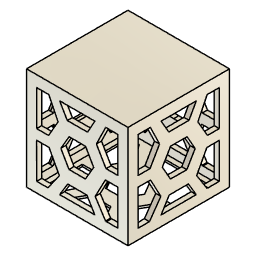
thermal and structural analaysis of cubesat (Autodesk Fusion 360 design; units mm, degrees)
part number: 2025-08-21-17-18-39-864
Autodesk Fusion 360 part; units mm, degrees
sketch "base sketch" plane through (0, 0, 0) normal (0, 0, 1) x (1, 0, 0)
  line L0 (25, -25) -> (-25, -25)
  line L1 (-25, -25) -> (-25, 25)
  line L2 (-25, 25) -> (25, 25)
  line L3 (25, 25) -> (25, -25)
  line L4 (14.1604, 2.5) -> (9.4273, 10.6474)
  line L5 (5.0651, 13.5136) -> (-4.9189, 13.4869)
  line L6 (-9.456, 10.6459) -> (-14.13, 2.5)
  line L7 (-4.6978, -13.5126) -> (4.7384, -13.4873)
  line L8 (8.827, -12.0049) -> (13.8516, -2.5)
  line L9 (8.0828, -0.0479) -> (4.0829, 6.9759)
  line L10 (4.0829, 6.9759) -> (-3.9999, 7.0238)
  line L11 (-3.9999, 7.0238) -> (-8.0828, 0.0479)
  line L12 (-8.0828, 0.0479) -> (-4.0829, -6.9759)
  line L13 (-4.0829, -6.9759) -> (3.9999, -7.0238)
  line L14 (3.9999, -7.0238) -> (8.0828, -0.0479)
  line L15 (-20, 20) -> (-14.435, 20)
  line L16 (-20, 20) -> (-20, 2.5)
  line L17 (-20, -20) -> (-14.435, -20)
  line L18 (-8.691, -20) -> (8.63, -20)
  line L19 (14.404, -20) -> (19.97, -20)
  line L20 (19.97, -20) -> (19.97, -2.5)
  line L21 (19.97, 2.5) -> (19.97, 20)
  line L22 (19.97, 20) -> (14.404, 20)
  line L23 (-8.661, 20) -> (8.66, 20)
  line L24 (8.66, 20) -> (5.0651, 13.5136)
  line L25 (-8.661, 20) -> (-4.9189, 13.4869)
  line L26 (-0.0005, 20) -> (1.3443, 20)
  line L27 (8.63, -20) -> (4.7384, -13.4873)
  line L28 (-8.691, -20) -> (-4.6978, -13.5126)
  line L29 (14, 20) -> (9.4273, 10.6474)
  line L30 (13.9944, 20) -> (16.5751, 20)
  line L31 (19.97, 2.5) -> (14.1604, 2.5)
  line L32 (19.97, -2.5) -> (13.8516, -2.5)
  arc A0 (13.9544, -19.9832) -> (14.404, -20) centre (14.404, -13.9776) ccw
  line L33 (8.827, -12.0049) -> (13.9544, -19.9832)
  line L34 (-14, 20) -> (-9.456, 10.6459)
  line L35 (-14.435, 20) -> (-14, 20)
  line L36 (-20, 2.5) -> (-14.13, 2.5)
  line L37 (-20.03, -20) -> (-20.03, -19.9999)
  line L38 (-20.03, -2.5001) -> (-20.03, -2.5)
  line L39 (-20.03, -20) -> (-20.03, -2.5)
  line L40 (-8.8138, -12.0049) -> (-14.435, -20)
  line L41 (-13.9188, -2.4938) -> (-20.0371, -2.4938)
  line L42 (-13.9188, -2.4938) -> (-8.8138, -12.0049)
  line L43 (-20.03, -2.5) -> (-20, -20)
  line L44 (-20.03, -20) -> (-14.435, -20)
  line L45 (-14.435, -20) -> (-8.8138, -12.0049)
  line L46 (-8.8138, -12.0049) -> (-13.9188, -2.4938)
  line L47 (-20.03, -2.5001) -> (-13.9188, -2.4938)
  line L48 (-13.9188, -2.4938) -> (-8.8138, -12.0049)
  line L49 (-8.8138, -12.0049) -> (-14.435, -20)
  line L50 (-14.435, -20) -> (-20, -20)
  dimension "d1" = 50
  dimension "d2" = 50
  dimension "d9" = 5.565
  dimension "d20" = 17.5
  dimension "d26" = 17.321
  dimension "d28" = 5.566
  dimension "d29" = 17.5
  dimension "d31" = 17.5
  dimension "d32" = 5.566
  dimension "d33" = 17.321
  dimension "d35" = 17.5
  dimension "d36" = 10.7512
  dimension "d37" = 17.5
  constraint horizontal L0
  constraint perpendicular L0 L1
  constraint parallel L0 L2
  constraint parallel L1 L3
  constraint perpendicular L15 L16
  constraint perpendicular L19 L20
  constraint perpendicular L21 L22
  constraint midpoint L23 L26.start
  constraint coincident L23 L26.end
  constraint coincident L22 L30.start
  constraint horizontal L30
  constraint perpendicular L21 L31
  constraint perpendicular L20 L32
  constraint tangent L19 A0
  constraint perpendicular L16 L36
  constraint coincident L38.start L37
  constraint collinear L37 L38
  constraint parallel L17 L44
  constraint perpendicular L39 L50
  measures "d1" distance of L1.end L2.end
  measures "d2" distance of L0.start L2.end
  measures "d9" distance of L15.start L15.end
  measures "d20" distance of L15.start L16.end
  measures "d26" distance of L18.start L18.end
  measures "d28" distance of L19.start L19.end
  measures "d29" distance of L19.end L20.end
  measures "d31" distance of L21.start L21.end
  measures "d32" distance of L21.end L22.end
  measures "d33" distance of L23.start L23.end
  measures "d35" distance of L37.start L38.end
  measures "d36" distance of L8.end L8.start
  measures "d37" distance of L38.end L37.start
extrude "Extrude1" add sketch "base sketch" along normal mid plane 50
sketch "Sketch14" plane through (25, 0, 0) normal (1, 0, 0) x (0, 1, 0)
  line L0 (25, -25) -> (25, 25)
  line L1 (25, 25) -> (-25, 25)
  line L2 (-25, 25) -> (-25, -25)
  line L3 (-25, -25) -> (25, -25)
  line L4 (-8.0828, 0.0479) -> (-4.0829, -6.9759)
  line L5 (8.827, -12.0049) -> (13.8516, -2.5)
  line L6 (-4.6978, -13.5126) -> (4.7384, -13.4873)
  line L7 (19.97, 2.5) -> (19.97, 20)
  line L8 (8.827, -12.0049) -> (13.9544, -19.9832)
  line L9 (8.0828, -0.0479) -> (4.0829, 6.9759)
  line L10 (3.9999, -7.0238) -> (8.0828, -0.0479)
  line L11 (-20, 20) -> (-20, 2.5)
  line L12 (13.9944, 20) -> (16.5751, 20)
  line L13 (-8.661, 20) -> (8.66, 20)
  line L14 (14, 20) -> (9.4273, 10.6474)
  line L15 (-8.691, -20) -> (8.63, -20)
  line L16 (-20, 20) -> (-14.435, 20)
  line L17 (8.63, -20) -> (4.7384, -13.4873)
  line L18 (-9.456, 10.6459) -> (-14.13, 2.5)
  line L19 (14.404, -20) -> (19.97, -20)
  line L20 (-14.435, 20) -> (-14, 20)
  line L21 (-4.0829, -6.9759) -> (3.9999, -7.0238)
  line L22 (14.1604, 2.5) -> (9.4273, 10.6474)
  line L23 (-0.0005, 20) -> (1.3443, 20)
  line L24 (19.97, -20) -> (19.97, -2.5)
  arc A0 (13.9544, -19.9832) -> (14.404, -20) centre (14.404, -13.9776) ccw
  line L25 (8.66, 20) -> (5.0651, 13.5136)
  line L26 (-3.9999, 7.0238) -> (-8.0828, 0.0479)
  line L27 (-13.9188, -2.4938) -> (-8.8138, -12.0049)
  line L28 (19.97, -2.5) -> (13.8516, -2.5)
  line L29 (-20.03, -2.5001) -> (-13.9188, -2.4938)
  line L30 (-20.03, -20) -> (-20.03, -2.5)
  line L31 (19.97, 20) -> (14.404, 20)
  line L32 (4.0829, 6.9759) -> (-3.9999, 7.0238)
  line L33 (-20, 2.5) -> (-14.13, 2.5)
  line L34 (-8.661, 20) -> (-4.9189, 13.4869)
  line L35 (19.97, 2.5) -> (14.1604, 2.5)
  line L36 (-8.8138, -12.0049) -> (-13.9188, -2.4938)
  line L37 (-14, 20) -> (-9.456, 10.6459)
  line L38 (5.0651, 13.5136) -> (-4.9189, 13.4869)
  line L39 (-13.9188, -2.4938) -> (-20.0371, -2.4938)
  line L40 (-8.8138, -12.0049) -> (-14.435, -20)
  line L41 (-20, -20) -> (-14.435, -20)
  line L42 (-20.03, -20) -> (-20.03, -19.9999)
  line L43 (-14.435, -20) -> (-8.8138, -12.0049)
  line L44 (-13.9188, -2.4938) -> (-8.8138, -12.0049)
  line L45 (-20.03, -20) -> (-14.435, -20)
  line L46 (-20.03, -2.5) -> (-20, -20)
  line L47 (-8.8138, -12.0049) -> (-14.435, -20)
  line L48 (-20.03, -2.5001) -> (-20.03, -2.5)
  line L49 (-8.691, -20) -> (-4.6978, -13.5126)
  line L50 (-14.435, -20) -> (-20, -20)
  dimension "d40" = 5.565
  dimension "d41" = 17.5
  dimension "d42" = 17.321
  dimension "d43" = 5.566
  dimension "d44" = 17.5
  dimension "d45" = 17.5
  dimension "d46" = 5.566
  dimension "d47" = 17.321
  dimension "d48" = 17.5
  dimension "d49" = 10.7512
  dimension "d50" = 17.5
  constraint perpendicular L11 L16
  constraint perpendicular L19 L24
  constraint perpendicular L7 L31
  constraint midpoint L23.start L13
  constraint coincident L23.end L13
  constraint coincident L12.start L31
  constraint horizontal L12
  constraint perpendicular L7 L35
  constraint perpendicular L24 L28
  constraint tangent L19 A0
  constraint perpendicular L11 L33
  constraint coincident L29.start L42
  constraint collinear L42 L48
  constraint parallel L41 L45
  constraint perpendicular L30 L50
  measures "d40" distance of L11.start L16.end
  measures "d41" distance of L11.end L11.start
  measures "d42" distance of L15.start L15.end
  measures "d43" distance of L19.start L19.end
  measures "d44" distance of L24.end L19.end
  measures "d45" distance of L7.start L7.end
  measures "d46" distance of L31.end L7.end
  measures "d47" distance of L13.start L13.end
  measures "d48" distance of L30.start L30.end
  measures "d49" distance of L5.start L5.end
  measures "d50" distance of L30.start L30.end
extrude "Extrude2" cut sketch "Sketch14" against normal blind 49 contours L4 L9 L10 L21 L26 L32 | L5 L8 L19 L24 A0 L28 | L6 L15 L17 L49 | L7 L12 L14 L22 L31 L35 | L11 L16 L18 L20 L33 L37 | L13 L23 L25 L34 L38 | L27 L29 L36 L40 L41 L43 L44 L45 L46 L47 L50
sketch "Sketch15" plane through (0, 25, 0) normal (0, 1, 0) x (-1, 0, 0)
  line L0 (25, -25) -> (25, 25)
  line L1 (25, 25) -> (-25, 25)
  line L2 (-25, 25) -> (-25, -25)
  line L3 (-25, -25) -> (25, -25)
  line L4 (-8.0828, 0.0479) -> (-4.0829, -6.9759)
  line L5 (8.827, -12.0049) -> (13.8516, -2.5)
  line L6 (-4.6978, -13.5126) -> (4.7384, -13.4873)
  line L7 (19.97, 2.5) -> (19.97, 20)
  line L8 (8.827, -12.0049) -> (13.9544, -19.9832)
  line L9 (8.0828, -0.0479) -> (4.0829, 6.9759)
  line L10 (3.9999, -7.0238) -> (8.0828, -0.0479)
  line L11 (-20, 20) -> (-20, 2.5)
  line L12 (13.9944, 20) -> (16.5751, 20)
  line L13 (-8.661, 20) -> (8.66, 20)
  line L14 (14, 20) -> (9.4273, 10.6474)
  line L15 (-8.691, -20) -> (8.63, -20)
  line L16 (-20, 20) -> (-14.435, 20)
  line L17 (8.63, -20) -> (4.7384, -13.4873)
  line L18 (-9.456, 10.6459) -> (-14.13, 2.5)
  line L19 (14.404, -20) -> (19.97, -20)
  line L20 (-14.435, 20) -> (-14, 20)
  line L21 (-4.0829, -6.9759) -> (3.9999, -7.0238)
  line L22 (14.1604, 2.5) -> (9.4273, 10.6474)
  line L23 (-0.0005, 20) -> (1.3443, 20)
  line L24 (19.97, -20) -> (19.97, -2.5)
  arc A0 (13.9544, -19.9832) -> (14.404, -20) centre (14.404, -13.9776) ccw
  line L25 (8.66, 20) -> (5.0651, 13.5136)
  line L26 (-3.9999, 7.0238) -> (-8.0828, 0.0479)
  line L27 (-13.9188, -2.4938) -> (-8.8138, -12.0049)
  line L28 (19.97, -2.5) -> (13.8516, -2.5)
  line L29 (-20.03, -2.5001) -> (-13.9188, -2.4938)
  line L30 (-20.03, -20) -> (-20.03, -2.5)
  line L31 (19.97, 20) -> (14.404, 20)
  line L32 (4.0829, 6.9759) -> (-3.9999, 7.0238)
  line L33 (-20, 2.5) -> (-14.13, 2.5)
  line L34 (-8.661, 20) -> (-4.9189, 13.4869)
  line L35 (19.97, 2.5) -> (14.1604, 2.5)
  line L36 (-8.8138, -12.0049) -> (-13.9188, -2.4938)
  line L37 (-14, 20) -> (-9.456, 10.6459)
  line L38 (5.0651, 13.5136) -> (-4.9189, 13.4869)
  line L39 (-13.9188, -2.4938) -> (-20.0371, -2.4938)
  line L40 (-8.8138, -12.0049) -> (-14.435, -20)
  line L41 (-20, -20) -> (-14.435, -20)
  line L42 (-20.03, -20) -> (-20.03, -19.9999)
  line L43 (-14.435, -20) -> (-8.8138, -12.0049)
  line L44 (-13.9188, -2.4938) -> (-8.8138, -12.0049)
  line L45 (-20.03, -20) -> (-14.435, -20)
  line L46 (-20.03, -2.5) -> (-20, -20)
  line L47 (-8.8138, -12.0049) -> (-14.435, -20)
  line L48 (-20.03, -2.5001) -> (-20.03, -2.5)
  line L49 (-8.691, -20) -> (-4.6978, -13.5126)
  line L50 (-14.435, -20) -> (-20, -20)
  dimension "d53" = 5.565
  dimension "d54" = 17.5
  dimension "d55" = 17.321
  dimension "d56" = 5.566
  dimension "d57" = 17.5
  dimension "d58" = 17.5
  dimension "d59" = 5.566
  dimension "d60" = 17.321
  dimension "d61" = 17.5
  dimension "d62" = 10.7512
  dimension "d63" = 17.5
  constraint perpendicular L11 L16
  constraint perpendicular L19 L24
  constraint perpendicular L7 L31
  constraint midpoint L23.start L13
  constraint coincident L23.end L13
  constraint coincident L12.start L31
  constraint horizontal L12
  constraint perpendicular L7 L35
  constraint perpendicular L24 L28
  constraint tangent L19 A0
  constraint perpendicular L11 L33
  constraint coincident L29.start L42
  constraint collinear L42 L48
  constraint parallel L41 L45
  constraint perpendicular L30 L50
  measures "d53" distance of L11.start L16.end
  measures "d54" distance of L11.end L11.start
  measures "d55" distance of L15.start L15.end
  measures "d56" distance of L19.start L19.end
  measures "d57" distance of L24.end L19.end
  measures "d58" distance of L7.start L7.end
  measures "d59" distance of L31.end L7.end
  measures "d60" distance of L13.start L13.end
  measures "d61" distance of L30.start L30.end
  measures "d62" distance of L5.start L5.end
  measures "d63" distance of L30.start L30.end
extrude "Extrude3" cut sketch "Sketch15" against normal blind 25 contours L4 L9 L10 L21 L26 L32 | L5 L8 L19 L24 A0 L28 | L6 L15 L17 L49 | L7 L12 L14 L22 L31 L35 | L11 L16 L18 L20 L33 L37 | L13 L23 L25 L34 L38 | L27 L29 L36 L40 L41 L43 L44 L45 L46 L47 L50
sketch "Sketch16" plane through (0, -25, 0) normal (0, -1, 0) x (1, 0, 0)
  line L0 (25, -25) -> (25, 25)
  line L1 (25, 25) -> (-25, 25)
  line L2 (-25, 25) -> (-25, -25)
  line L3 (-25, -25) -> (25, -25)
  line L4 (-8.0828, 0.0479) -> (-4.0829, -6.9759)
  line L5 (8.827, -12.0049) -> (13.8516, -2.5)
  line L6 (-4.6978, -13.5126) -> (4.7384, -13.4873)
  line L7 (19.97, 2.5) -> (19.97, 20)
  line L8 (8.827, -12.0049) -> (13.9544, -19.9832)
  line L9 (8.0828, -0.0479) -> (4.0829, 6.9759)
  line L10 (3.9999, -7.0238) -> (8.0828, -0.0479)
  line L11 (-20, 20) -> (-20, 2.5)
  line L12 (13.9944, 20) -> (16.5751, 20)
  line L13 (-8.661, 20) -> (8.66, 20)
  line L14 (14, 20) -> (9.4273, 10.6474)
  line L15 (-8.691, -20) -> (8.63, -20)
  line L16 (-20, 20) -> (-14.435, 20)
  line L17 (8.63, -20) -> (4.7384, -13.4873)
  line L18 (-9.456, 10.6459) -> (-14.13, 2.5)
  line L19 (14.404, -20) -> (19.97, -20)
  line L20 (-14.435, 20) -> (-14, 20)
  line L21 (-4.0829, -6.9759) -> (3.9999, -7.0238)
  line L22 (14.1604, 2.5) -> (9.4273, 10.6474)
  line L23 (-0.0005, 20) -> (1.3443, 20)
  line L24 (19.97, -20) -> (19.97, -2.5)
  arc A0 (13.9544, -19.9832) -> (14.404, -20) centre (14.404, -13.9776) ccw
  line L25 (8.66, 20) -> (5.0651, 13.5136)
  line L26 (-3.9999, 7.0238) -> (-8.0828, 0.0479)
  line L27 (-13.9188, -2.4938) -> (-8.8138, -12.0049)
  line L28 (19.97, -2.5) -> (13.8516, -2.5)
  line L29 (-20.03, -2.5001) -> (-13.9188, -2.4938)
  line L30 (-20.03, -20) -> (-20.03, -2.5)
  line L31 (19.97, 20) -> (14.404, 20)
  line L32 (4.0829, 6.9759) -> (-3.9999, 7.0238)
  line L33 (-20, 2.5) -> (-14.13, 2.5)
  line L34 (-8.661, 20) -> (-4.9189, 13.4869)
  line L35 (19.97, 2.5) -> (14.1604, 2.5)
  line L36 (-8.8138, -12.0049) -> (-13.9188, -2.4938)
  line L37 (-14, 20) -> (-9.456, 10.6459)
  line L38 (5.0651, 13.5136) -> (-4.9189, 13.4869)
  line L39 (-13.9188, -2.4938) -> (-20.0371, -2.4938)
  line L40 (-8.8138, -12.0049) -> (-14.435, -20)
  line L41 (-20, -20) -> (-14.435, -20)
  line L42 (-20.03, -20) -> (-20.03, -19.9999)
  line L43 (-14.435, -20) -> (-8.8138, -12.0049)
  line L44 (-13.9188, -2.4938) -> (-8.8138, -12.0049)
  line L45 (-20.03, -20) -> (-14.435, -20)
  line L46 (-20.03, -2.5) -> (-20, -20)
  line L47 (-8.8138, -12.0049) -> (-14.435, -20)
  line L48 (-20.03, -2.5001) -> (-20.03, -2.5)
  line L49 (-8.691, -20) -> (-4.6978, -13.5126)
  line L50 (-14.435, -20) -> (-20, -20)
  dimension "d66" = 5.565
  dimension "d67" = 17.5
  dimension "d68" = 17.321
  dimension "d69" = 5.566
  dimension "d70" = 17.5
  dimension "d71" = 17.5
  dimension "d72" = 5.566
  dimension "d73" = 17.321
  dimension "d74" = 17.5
  dimension "d75" = 10.7512
  dimension "d76" = 17.5
  constraint perpendicular L11 L16
  constraint perpendicular L19 L24
  constraint perpendicular L7 L31
  constraint midpoint L23.start L13
  constraint coincident L23.end L13
  constraint coincident L12.start L31
  constraint horizontal L12
  constraint perpendicular L7 L35
  constraint perpendicular L24 L28
  constraint tangent L19 A0
  constraint perpendicular L11 L33
  constraint coincident L29.start L42
  constraint collinear L42 L48
  constraint parallel L41 L45
  constraint perpendicular L30 L50
  measures "d66" distance of L11.start L16.end
  measures "d67" distance of L11.end L11.start
  measures "d68" distance of L15.start L15.end
  measures "d69" distance of L19.start L19.end
  measures "d70" distance of L24.end L19.end
  measures "d71" distance of L7.start L7.end
  measures "d72" distance of L31.end L7.end
  measures "d73" distance of L13.start L13.end
  measures "d74" distance of L30.start L30.end
  measures "d75" distance of L5.start L5.end
  measures "d76" distance of L30.start L30.end
extrude "Extrude4" cut sketch "Sketch16" against normal blind 50 contours L4 L9 L10 L21 L26 L32 | L5 L8 L19 L24 A0 L28 | L6 L15 L17 L49 | L7 L12 L14 L22 L31 L35 | L11 L16 L18 L20 L33 L37 | L13 L23 L25 L34 L38 | L27 L29 L36 L40 L41 L43 L44 L45 L46 L47 L50
sketch "Sketch17" plane through (-25, 0, 0) normal (-1, 0, 0) x (0, -1, 0)
  line L0 (25, -25) -> (25, 25)
  line L1 (25, 25) -> (-25, 25)
  line L2 (-25, 25) -> (-25, -25)
  line L3 (-25, -25) -> (25, -25)
  line L4 (-8.0828, 0.0479) -> (-4.0829, -6.9759)
  line L5 (8.827, -12.0049) -> (13.8516, -2.5)
  line L6 (-4.6978, -13.5126) -> (4.7384, -13.4873)
  line L7 (19.97, 2.5) -> (19.97, 20)
  line L8 (8.827, -12.0049) -> (13.9544, -19.9832)
  line L9 (8.0828, -0.0479) -> (4.0829, 6.9759)
  line L10 (3.9999, -7.0238) -> (8.0828, -0.0479)
  line L11 (-20, 20) -> (-20, 2.5)
  line L12 (13.9944, 20) -> (16.5751, 20)
  line L13 (-8.661, 20) -> (8.66, 20)
  line L14 (14, 20) -> (9.4273, 10.6474)
  line L15 (-8.691, -20) -> (8.63, -20)
  line L16 (-20, 20) -> (-14.435, 20)
  line L17 (8.63, -20) -> (4.7384, -13.4873)
  line L18 (-9.456, 10.6459) -> (-14.13, 2.5)
  line L19 (14.404, -20) -> (19.97, -20)
  line L20 (-14.435, 20) -> (-14, 20)
  line L21 (-4.0829, -6.9759) -> (3.9999, -7.0238)
  line L22 (14.1604, 2.5) -> (9.4273, 10.6474)
  line L23 (-0.0005, 20) -> (1.3443, 20)
  line L24 (19.97, -20) -> (19.97, -2.5)
  arc A0 (13.9544, -19.9832) -> (14.404, -20) centre (14.404, -13.9776) ccw
  line L25 (8.66, 20) -> (5.0651, 13.5136)
  line L26 (-3.9999, 7.0238) -> (-8.0828, 0.0479)
  line L27 (-13.9188, -2.4938) -> (-8.8138, -12.0049)
  line L28 (19.97, -2.5) -> (13.8516, -2.5)
  line L29 (-20.03, -2.5001) -> (-13.9188, -2.4938)
  line L30 (-20.03, -20) -> (-20.03, -2.5)
  line L31 (19.97, 20) -> (14.404, 20)
  line L32 (4.0829, 6.9759) -> (-3.9999, 7.0238)
  line L33 (-20, 2.5) -> (-14.13, 2.5)
  line L34 (-8.661, 20) -> (-4.9189, 13.4869)
  line L35 (19.97, 2.5) -> (14.1604, 2.5)
  line L36 (-8.8138, -12.0049) -> (-13.9188, -2.4938)
  line L37 (-14, 20) -> (-9.456, 10.6459)
  line L38 (5.0651, 13.5136) -> (-4.9189, 13.4869)
  line L39 (-13.9188, -2.4938) -> (-20.0371, -2.4938)
  line L40 (-8.8138, -12.0049) -> (-14.435, -20)
  line L41 (-20, -20) -> (-14.435, -20)
  line L42 (-20.03, -20) -> (-20.03, -19.9999)
  line L43 (-14.435, -20) -> (-8.8138, -12.0049)
  line L44 (-13.9188, -2.4938) -> (-8.8138, -12.0049)
  line L45 (-20.03, -20) -> (-14.435, -20)
  line L46 (-20.03, -2.5) -> (-20, -20)
  line L47 (-8.8138, -12.0049) -> (-14.435, -20)
  line L48 (-20.03, -2.5001) -> (-20.03, -2.5)
  line L49 (-8.691, -20) -> (-4.6978, -13.5126)
  line L50 (-14.435, -20) -> (-20, -20)
  dimension "d79" = 5.565
  dimension "d80" = 17.5
  dimension "d81" = 17.321
  dimension "d82" = 5.566
  dimension "d83" = 17.5
  dimension "d84" = 17.5
  dimension "d85" = 5.566
  dimension "d86" = 17.321
  dimension "d87" = 17.5
  dimension "d88" = 10.7512
  dimension "d89" = 17.5
  constraint perpendicular L11 L16
  constraint perpendicular L19 L24
  constraint perpendicular L7 L31
  constraint midpoint L23.start L13
  constraint coincident L23.end L13
  constraint coincident L12.start L31
  constraint horizontal L12
  constraint perpendicular L7 L35
  constraint perpendicular L24 L28
  constraint tangent L19 A0
  constraint perpendicular L11 L33
  constraint coincident L29.start L42
  constraint collinear L42 L48
  constraint parallel L41 L45
  constraint perpendicular L30 L50
  measures "d79" distance of L11.start L16.end
  measures "d80" distance of L11.end L11.start
  measures "d81" distance of L15.start L15.end
  measures "d82" distance of L19.start L19.end
  measures "d83" distance of L24.end L19.end
  measures "d84" distance of L7.start L7.end
  measures "d85" distance of L31.end L7.end
  measures "d86" distance of L13.start L13.end
  measures "d87" distance of L30.start L30.end
  measures "d88" distance of L5.start L5.end
  measures "d89" distance of L30.start L30.end
extrude "Extrude5" cut sketch "Sketch17" against normal blind 1 contours L4 L9 L10 L21 L26 L32 | L5 L8 L19 L24 A0 L28 | L6 L15 L17 L49 | L7 L12 L14 L22 L31 L35 | L11 L16 L18 L20 L33 L37 | L13 L23 L25 L34 L38 | L27 L29 L36 L40 L41 L43 L44 L45 L46 L47 L50
sketch "Sketch18" plane through (0, 0, 25) normal (0, 0, 1) x (-1, 0, 0)
  line L0 (-13.9544, 19.9832) -> (-8.827, 12.0049)
  line L1 (-8.827, 12.0049) -> (-13.8516, 2.5)
  line L2 (-13.8516, 2.5) -> (-19.97, 2.5)
  line L3 (-19.97, 2.5) -> (-19.97, 20)
  line L4 (-19.97, 20) -> (-14.404, 20)
  arc A0 (-13.9544, 19.9832) -> (-14.404, 20) centre (-14.404, 13.9776) ccw
  line L5 (-8.0828, 0.0479) -> (-3.9999, 7.0238)
  line L6 (-3.9999, 7.0238) -> (4.0829, 6.9759)
  line L7 (4.0829, 6.9759) -> (8.0828, -0.0479)
  line L8 (8.0828, -0.0479) -> (3.9999, -7.0238)
  line L9 (3.9999, -7.0238) -> (-4.0829, -6.9759)
  line L10 (-4.0829, -6.9759) -> (-8.0828, 0.0479)
  line L11 (8.8138, 12.0049) -> (14.435, 20)
  line L12 (14.435, 20) -> (20.03, 20)
  line L13 (20.03, 20) -> (20.03, 2.5001)
  line L14 (20.03, 2.5001) -> (13.9188, 2.4938)
  line L15 (13.9188, 2.4938) -> (8.8138, 12.0049)
  line L16 (-4.7384, 13.4873) -> (-8.63, 20)
  line L17 (-8.63, 20) -> (8.691, 20)
  line L18 (8.691, 20) -> (4.6978, 13.5126)
  line L19 (4.6978, 13.5126) -> (-4.7384, 13.4873)
  line L20 (20, -2.5) -> (20, -20)
  line L21 (20, -20) -> (14.435, -20)
  line L22 (14.435, -20) -> (14, -20)
  line L23 (14, -20) -> (9.456, -10.6459)
  line L24 (9.456, -10.6459) -> (14.13, -2.5)
  line L25 (14.13, -2.5) -> (20, -2.5)
  line L26 (4.9189, -13.4869) -> (8.661, -20)
  line L27 (8.661, -20) -> (-8.66, -20)
  line L28 (-8.66, -20) -> (-5.0651, -13.5136)
  line L29 (-5.0651, -13.5136) -> (4.9189, -13.4869)
  line L30 (-14, -20) -> (-19.97, -20)
  line L31 (-19.97, -20) -> (-19.97, -2.5)
  line L32 (-19.97, -2.5) -> (-14.1604, -2.5)
  line L33 (-14.1604, -2.5) -> (-9.4273, -10.6474)
  line L34 (-9.4273, -10.6474) -> (-14, -20)
  line L35 (-25, -25) -> (25, -25)
  line L36 (25, -25) -> (25, 25)
  line L37 (25, 25) -> (-25, 25)
  line L38 (-25, 25) -> (-25, -25)
  line L39 (-25, 25) -> (25, 25)
  line L40 (25, 25) -> (25, -25)
  line L41 (25, -25) -> (-25, -25)
  line L42 (-25, -25) -> (-25, 25)
  line L43 (-25, 25) -> (25, -25) construction
  line L44 (25, 25) -> (-25, -25) construction
  constraint horizontal L39
  constraint perpendicular L39 L40
  constraint parallel L39 L41
  constraint parallel L40 L42
  constraint coincident L43 origin
  constraint coincident L44 origin
  constraint coincident L37.end L38.start
extrude "Extrude6" add sketch "Sketch18" along normal blind 0.5 contours L0 L1 L2 L3 L4 A0 | L5 L6 L7 L8 L9 L10 | L11 L12 L13 L14 L15 | L16 L17 L18 L19 | L20 L21 L22 L23 L24 L25 | L26 L27 L28 L29 | L30 L31 L32 L33 L34 | L35 L36 L37 L38 L39 L40 L41 L42
sketch "Sketch19" plane through (25, 0, 0) normal (1, 0, 0) x (0, 1, 0)
sketch "Sketch20" plane through (0, 0, -25) normal (0, 0, -1) x (1, 0, 0)
  line L0 (8.827, 12.0049) -> (13.9544, 19.9832)
  arc A0 (14.404, 20) -> (13.9544, 19.9832) centre (14.404, 13.9776) ccw
  line L1 (14.404, 20) -> (19.97, 20)
  line L2 (19.97, 20) -> (19.97, 2.5)
  line L3 (19.97, 2.5) -> (13.8516, 2.5)
  line L4 (13.8516, 2.5) -> (8.827, 12.0049)
  line L5 (3.9999, 7.0238) -> (8.0828, 0.0479)
  line L6 (8.0828, 0.0479) -> (4.0829, -6.9759)
  line L7 (4.0829, -6.9759) -> (-3.9999, -7.0238)
  line L8 (-3.9999, -7.0238) -> (-8.0828, -0.0479)
  line L9 (-8.0828, -0.0479) -> (-4.0829, 6.9759)
  line L10 (-4.0829, 6.9759) -> (3.9999, 7.0238)
  line L11 (-14.435, 20) -> (-8.8138, 12.0049)
  line L12 (-8.8138, 12.0049) -> (-13.9188, 2.4938)
  line L13 (-13.9188, 2.4938) -> (-20.03, 2.5001)
  line L14 (-20.03, 2.5001) -> (-20.03, 20)
  line L15 (-20.03, 20) -> (-14.435, 20)
  line L16 (8.63, 20) -> (4.7384, 13.4873)
  line L17 (4.7384, 13.4873) -> (-4.6978, 13.5126)
  line L18 (-4.6978, 13.5126) -> (-8.691, 20)
  line L19 (-8.691, 20) -> (8.63, 20)
  line L20 (-20, -20) -> (-20, -2.5)
  line L21 (-20, -2.5) -> (-14.13, -2.5)
  line L22 (-14.13, -2.5) -> (-9.456, -10.6459)
  line L23 (-9.456, -10.6459) -> (-14, -20)
  line L24 (-14, -20) -> (-14.435, -20)
  line L25 (-14.435, -20) -> (-20, -20)
  line L26 (-8.661, -20) -> (-4.9189, -13.4869)
  line L27 (-4.9189, -13.4869) -> (5.0651, -13.5136)
  line L28 (5.0651, -13.5136) -> (8.66, -20)
  line L29 (8.66, -20) -> (-8.661, -20)
  line L30 (19.97, -20) -> (14, -20)
  line L31 (14, -20) -> (9.4273, -10.6474)
  line L32 (9.4273, -10.6474) -> (14.1604, -2.5)
  line L33 (14.1604, -2.5) -> (19.97, -2.5)
  line L34 (19.97, -2.5) -> (19.97, -20)
  line L35 (-25, -25) -> (25, -25)
  line L36 (25, -25) -> (25, 25)
  line L37 (25, 25) -> (-25, 25)
  line L38 (-25, 25) -> (-25, -25)
  line L39 (22.5, 22.5) -> (-22.5, 22.5)
  line L40 (-22.5, 22.5) -> (-22.5, -22.5)
  line L41 (-22.5, -22.5) -> (22.5, -22.5)
  line L42 (22.5, -22.5) -> (22.5, 22.5)
  line L43 (22.5, 22.5) -> (-22.5, -22.5) construction
  line L44 (-22.5, 22.5) -> (22.5, -22.5) construction
  dimension "d94" = 45
  dimension "d95" = 45
  constraint horizontal L39
  constraint perpendicular L39 L40
  constraint parallel L39 L41
  constraint parallel L40 L42
  constraint coincident L43 origin
  constraint coincident L44 origin
  measures "d94" distance of L40.end L41.end
  measures "d95" distance of L39.end L40.end
ref_plane "WorkPlane1" through (0, 0, -24) normal (0, 0, -1) x (1, 0, 0)
extrude "Extrude7" cut sketch "Sketch20" against normal blind 48 contours L39 L40 L41 L42
sketch "Sketch21" plane through (25, 0, 0) normal (1, 0, 0) x (0, 1, 0)
sketch "Sketch22" plane through (0, 0, -25) normal (0, 0, -1) x (1, 0, 0)
  line L0 (-22.5, 22.5) -> (22.5, 22.5)
  line L1 (22.5, 22.5) -> (22.5, -22.5)
  line L2 (22.5, -22.5) -> (-22.5, -22.5)
  line L3 (-22.5, -22.5) -> (-22.5, 22.5)
  line L4 (-25, -25) -> (25, -25)
  line L5 (25, -25) -> (25, 25)
  line L6 (25, 25) -> (-25, 25)
  line L7 (-25, 25) -> (-25, -25)
  line L8 (25, -25) -> (-25, -25)
  line L9 (-25, -25) -> (-25, 25)
  line L10 (-25, 25) -> (25, 25)
  line L11 (25, 25) -> (25, -25)
  line L12 (25, -25) -> (-25, 25) construction
  line L13 (-25, -25) -> (25, 25) construction
  constraint horizontal L8
  constraint perpendicular L8 L9
  constraint parallel L8 L10
  constraint parallel L9 L11
  constraint coincident L12 origin
  constraint coincident L13 origin
  constraint coincident L4.end L5.start
sketch "Sketch23" plane through (0, 0, -25) normal (0, 0, -1) x (1, 0, 0)
sketch "Sketch24" plane through (0, 0, 0) normal (0, 0, 1) x (1, 0, 0)
  line L0 (-25, -25) -> (25, -25)
  line L1 (25, -25) -> (25, 25)
  line L2 (25, 25) -> (-25, 25)
  line L3 (-25, 25) -> (-25, -25)
  line L4 (-25, -25) -> (25, 25) construction
  line L5 (25, -25) -> (-25, 25) construction
  line L6 (19.97, -2.5) -> (13.8516, -2.5)
  line L7 (-13.9188, -2.4938) -> (-8.8138, -12.0049)
  line L8 (-20.03, -20) -> (-20.03, -19.9999)
  line L9 (-13.9188, -2.4938) -> (-20.0371, -2.4938)
  line L10 (-0.0005, 20) -> (1.3443, 20)
  line L11 (-20, -20) -> (-14.435, -20)
  line L12 (-8.8138, -12.0049) -> (-14.435, -20)
  arc A0 (13.9544, -19.9832) -> (14.404, -20) centre (14.404, -13.9776) ccw
  line L13 (8.63, -20) -> (4.7384, -13.4873)
  line L14 (-3.9999, 7.0238) -> (-8.0828, 0.0479)
  line L15 (19.97, -20) -> (19.97, -2.5)
  line L16 (14, 20) -> (9.4273, 10.6474)
  line L17 (-8.691, -20) -> (-4.6978, -13.5126)
  line L18 (14.1604, 2.5) -> (9.4273, 10.6474)
  line L19 (-8.661, 20) -> (-4.9189, 13.4869)
  line L20 (-9.456, 10.6459) -> (-14.13, 2.5)
  line L21 (-20, 20) -> (-20, 2.5)
  line L22 (-14.435, 20) -> (-14, 20)
  line L23 (8.66, 20) -> (5.0651, 13.5136)
  line L24 (-20.03, -2.5001) -> (-13.9188, -2.4938)
  line L25 (-8.8138, -12.0049) -> (-14.435, -20)
  line L26 (-14.435, -20) -> (-8.8138, -12.0049)
  line L27 (8.827, -12.0049) -> (13.9544, -19.9832)
  line L28 (-8.661, 20) -> (8.66, 20)
  line L29 (-14.435, -20) -> (-20, -20)
  line L30 (8.827, -12.0049) -> (13.8516, -2.5)
  line L31 (4.0829, 6.9759) -> (-3.9999, 7.0238)
  line L32 (13.9944, 20) -> (16.5751, 20)
  line L33 (14.404, -20) -> (19.97, -20)
  line L34 (19.97, 2.5) -> (19.97, 20)
  line L35 (5.0651, 13.5136) -> (-4.9189, 13.4869)
  line L36 (8.0828, -0.0479) -> (4.0829, 6.9759)
  line L37 (-8.0828, 0.0479) -> (-4.0829, -6.9759)
  line L38 (-4.0829, -6.9759) -> (3.9999, -7.0238)
  line L39 (-4.6978, -13.5126) -> (4.7384, -13.4873)
  line L40 (-8.691, -20) -> (8.63, -20)
  line L41 (3.9999, -7.0238) -> (8.0828, -0.0479)
  line L42 (-20, 20) -> (-14.435, 20)
  line L43 (-13.9188, -2.4938) -> (-8.8138, -12.0049)
  line L44 (-20, 2.5) -> (-14.13, 2.5)
  line L45 (-20.03, -20) -> (-20.03, -2.5)
  line L46 (-14, 20) -> (-9.456, 10.6459)
  line L47 (-20.03, -2.5001) -> (-20.03, -2.5)
  line L48 (-20.03, -20) -> (-14.435, -20)
  line L49 (19.97, 2.5) -> (14.1604, 2.5)
  line L50 (-20.03, -2.5) -> (-20, -20)
  line L51 (19.97, 20) -> (14.404, 20)
  line L52 (-8.8138, -12.0049) -> (-13.9188, -2.4938)
  dimension "d99" = 5.565
  dimension "d100" = 17.5
  dimension "d101" = 17.321
  dimension "d102" = 5.566
  dimension "d103" = 17.5
  dimension "d104" = 17.5
  dimension "d105" = 5.566
  dimension "d106" = 17.321
  dimension "d107" = 17.5
  dimension "d108" = 10.7512
  dimension "d109" = 17.5
  constraint horizontal L0
  constraint perpendicular L0 L1
  constraint parallel L0 L2
  constraint parallel L1 L3
  constraint coincident L4 origin
  constraint coincident L5 origin
  constraint perpendicular L21 L42
  constraint perpendicular L15 L33
  constraint perpendicular L34 L51
  constraint midpoint L10.start L28
  constraint coincident L10.end L28
  constraint coincident L32.start L51
  constraint horizontal L32
  constraint perpendicular L34 L49
  constraint perpendicular L6 L15
  constraint tangent A0 L33
  constraint perpendicular L21 L44
  constraint coincident L24.start L8
  constraint collinear L8 L47
  constraint parallel L11 L48
  constraint perpendicular L29 L45
  measures "d99" distance of L21.start L22.start
  measures "d100" distance of L21.end L21.start
  measures "d101" distance of L17.start L13.start
  measures "d102" distance of L15.start A0.end
  measures "d103" distance of L15.start L6.start
  measures "d104" distance of L34.end L34.start
  measures "d105" distance of L51.end L34.end
  measures "d106" distance of L19.start L23.start
  measures "d107" distance of L45.end L8.start
  measures "d108" distance of L27.start L6.end
  measures "d109" distance of L8.start L45.end
sketch "Sketch25" plane through (0, 0, 0) normal (0, 0, 1) x (1, 0, 0)
  line L0 (-25, -25) -> (25, -25)
  line L1 (25, -25) -> (25, 25)
  line L2 (25, 25) -> (-25, 25)
  line L3 (-25, 25) -> (-25, -25)
  line L4 (-25, -25) -> (25, 25) construction
  line L5 (25, -25) -> (-25, 25) construction
  constraint horizontal L0
  constraint perpendicular L0 L1
  constraint parallel L0 L2
  constraint parallel L1 L3
  constraint coincident L4 origin
  constraint coincident L5 origin
sketch "Sketch26" plane through (0, 0, -25) normal (0, 0, -1) x (1, 0, 0)
  line L0 (-22.5, 22.5) -> (22.5, 22.5)
  line L1 (22.5, 22.5) -> (22.5, -22.5)
  line L2 (22.5, -22.5) -> (-22.5, -22.5)
  line L3 (-22.5, -22.5) -> (-22.5, 22.5)
  line L4 (-25, -25) -> (25, -25)
  line L5 (25, -25) -> (25, 25)
  line L6 (25, 25) -> (-25, 25)
  line L7 (-25, 25) -> (-25, -25)
  line L8 (25, -25) -> (-25, -25)
  line L9 (-25, -25) -> (-25, 25)
  line L10 (-25, 25) -> (25, 25)
  line L11 (25, 25) -> (25, -25)
  line L12 (19.97, -2.5) -> (13.8516, -2.5)
  line L13 (-13.9188, -2.4938) -> (-8.8138, -12.0049)
  line L14 (-20.03, -20) -> (-20.03, -19.9999)
  line L15 (-13.9188, -2.4938) -> (-20.0371, -2.4938)
  line L16 (-0.0005, 20) -> (1.3443, 20)
  line L17 (-20, -20) -> (-14.435, -20)
  line L18 (-8.8138, -12.0049) -> (-14.435, -20)
  arc A0 (13.9544, -19.9832) -> (14.404, -20) centre (14.404, -13.9776) ccw
  line L19 (8.63, -20) -> (4.7384, -13.4873)
  line L20 (-3.9999, 7.0238) -> (-8.0828, 0.0479)
  line L21 (19.97, -20) -> (19.97, -2.5)
  line L22 (14, 20) -> (9.4273, 10.6474)
  line L23 (-8.691, -20) -> (-4.6978, -13.5126)
  line L24 (14.1604, 2.5) -> (9.4273, 10.6474)
  line L25 (-8.661, 20) -> (-4.9189, 13.4869)
  line L26 (-9.456, 10.6459) -> (-14.13, 2.5)
  line L27 (-20, 20) -> (-20, 2.5)
  line L28 (-14.435, 20) -> (-14, 20)
  line L29 (8.66, 20) -> (5.0651, 13.5136)
  line L30 (-20.03, -2.5001) -> (-13.9188, -2.4938)
  line L31 (-8.8138, -12.0049) -> (-14.435, -20)
  line L32 (-14.435, -20) -> (-8.8138, -12.0049)
  line L33 (8.827, -12.0049) -> (13.9544, -19.9832)
  line L34 (-8.661, 20) -> (8.66, 20)
  line L35 (-14.435, -20) -> (-20, -20)
  line L36 (8.827, -12.0049) -> (13.8516, -2.5)
  line L37 (4.0829, 6.9759) -> (-3.9999, 7.0238)
  line L38 (13.9944, 20) -> (16.5751, 20)
  line L39 (14.404, -20) -> (19.97, -20)
  line L40 (19.97, 2.5) -> (19.97, 20)
  line L41 (5.0651, 13.5136) -> (-4.9189, 13.4869)
  line L42 (8.0828, -0.0479) -> (4.0829, 6.9759)
  line L43 (-8.0828, 0.0479) -> (-4.0829, -6.9759)
  line L44 (-4.0829, -6.9759) -> (3.9999, -7.0238)
  line L45 (-4.6978, -13.5126) -> (4.7384, -13.4873)
  line L46 (-8.691, -20) -> (8.63, -20)
  line L47 (3.9999, -7.0238) -> (8.0828, -0.0479)
  line L48 (-20, 20) -> (-14.435, 20)
  line L49 (-13.9188, -2.4938) -> (-8.8138, -12.0049)
  line L50 (-20, 2.5) -> (-14.13, 2.5)
  line L51 (-20.03, -20) -> (-20.03, -2.5)
  line L52 (-14, 20) -> (-9.456, 10.6459)
  line L53 (-20.03, -2.5001) -> (-20.03, -2.5)
  line L54 (-20.03, -20) -> (-14.435, -20)
  line L55 (19.97, 2.5) -> (14.1604, 2.5)
  line L56 (-20.03, -2.5) -> (-20, -20)
  line L57 (19.97, 20) -> (14.404, 20)
  line L58 (-8.8138, -12.0049) -> (-13.9188, -2.4938)
  dimension "d110" = 5.565
  dimension "d111" = 17.5
  dimension "d112" = 17.321
  dimension "d113" = 5.566
  dimension "d114" = 17.5
  dimension "d115" = 17.5
  dimension "d116" = 5.566
  dimension "d117" = 17.321
  dimension "d118" = 17.5
  dimension "d119" = 10.7512
  dimension "d120" = 17.5
  constraint horizontal L8
  constraint vertical L9
  constraint horizontal L10
  constraint vertical L11
  constraint coincident L6.end L7.start
  constraint coincident L4.end L5.start
  constraint perpendicular L27 L48
  constraint perpendicular L21 L39
  constraint perpendicular L40 L57
  constraint midpoint L16.start L34
  constraint coincident L16.end L34
  constraint coincident L38.start L57
  constraint horizontal L38
  constraint perpendicular L40 L55
  constraint perpendicular L12 L21
  constraint tangent A0 L39
  constraint perpendicular L27 L50
  constraint coincident L30.start L14
  constraint collinear L14 L53
  constraint parallel L17 L54
  constraint perpendicular L35 L51
  measures "d110" distance of L27.start L28.start
  measures "d111" distance of L27.end L27.start
  measures "d112" distance of L23.start L19.start
  measures "d113" distance of L21.start A0.end
  measures "d114" distance of L21.start L12.start
  measures "d115" distance of L40.end L40.start
  measures "d116" distance of L57.end L40.end
  measures "d117" distance of L25.start L29.start
  measures "d118" distance of L51.end L14.start
  measures "d119" distance of L33.start L12.end
  measures "d120" distance of L14.start L51.end
extrude "Extrude8" add sketch "Sketch26" against normal blind 1 contours L0 L1 L2 L3
